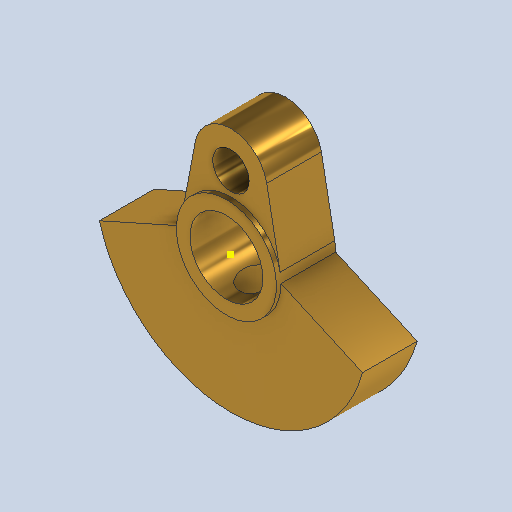
# Autodesk Inventor part: KURBEL PART 8
Saved by Autodesk Inventor 2022 (Build 260153000, 153)
## iProperties
Created: 2020-07-02
Part Number: KURBEL PART 8
Material: Generic
Document SubType Name: Modeling
Designer: Smit Ambardekar
Density: 1 g/cm^3
Appearance: Default
Author: Smit Ambardekar
Autodesk Inventor part; units mm, degrees
ref_plane "YZ Plane" through (0, 0, 0) normal (1, 0, 0) x (0, 1, 0)
ref_plane "XZ Plane" through (0, 0, 0) normal (0, 1, 0) x (-1, 0, 0)
sketch "Sketch1" plane through (0, 0, 0) normal (0, 0, 1) x (1, 0, 0)
  arc A0 (-14.4568, -4) -> (14.4568, -4) centre (0, 0) ccw
  circle A1 centre (0, 0) radius 5.5
  line L0 (0, 0) -> (0, -4)
  line L1 (-5.5, 0) -> (-14.4568, -4)
  line L2 (5.5, 0) -> (14.4568, -4)
  line L3 (0, 0) -> (0, 8)
  circle A2 centre (0, 8) radius 2
  line L4 (-5.4025, 1.0312) -> (-3.9291, 8.75)
  line L5 (3.9291, 8.75) -> (5.4025, 1.0313)
  arc A3 (3.9291, 8.75) -> (-3.9291, 8.75) centre (0, 8) ccw
  line L6 (-2, 14.8661) -> (2, 14.8661)
  line L7 (2, 14.8661) -> (2, -14.8661)
  line L8 (2, -14.8661) -> (-2, -14.8661)
  line L9 (-2, -14.8661) -> (-2, 14.8661)
  line L10 (-2, 14.8661) -> (2, -14.8661) construction
  line L11 (2, 14.8661) -> (-2, -14.8661) construction
  dimension "d0" = 30
  dimension "d1" = 11
  dimension "d2" = 4
  dimension "d3" = 8
  dimension "d4" = 4
  constraints: 24 end point, 9 point on circle, 4 centre point, 4 coincident, 4 tangent, 2 midpoint, 2 parallel, 2 vertical, 1 horizontal, 1 perpendicular
  measures "d0" diameter of A0
  measures "d1" diameter of A1
  measures "d2" distance of L0.start L0.end
  measures "d3" distance of L0.start L3.end
  measures "d4" diameter of A2
extrude "Extrusion1" add sketch "Sketch1" along normal blind 6 contours L1 A1 L9 A0 | L8 A0 | L9 A1 L7 L8 | A1 L9 | L7 A1 L2 A0 | L9 A1 L7 | L4 A3 L9 A1 | L7 A1 | L9 A2 L3 A1 | L7 A3 L5 A1 | A1 L3 A2 L7 | L9 A3 L7 A2
sketch "Sketch2" plane through (0, 0, 6) normal (0, 0, 1) x (1, 0, 0)
  arc A0 (5.5, 0) -> (5.4025, 1.0313) centre (0, 0) ccw projected
  circle A1 centre (0, 0) radius 5.5
  point P0 (5.4025, 1.0313)
  constraints: 1 coincident, 3 other
extrude "Extrusion2" add sketch "Sketch2" along normal blind 0.5
sketch "Sketch3" plane through (0, 0, 6.5) normal (0, 0, 1) x (1, 0, 0)
  point P0 (0, 0)
hole "Hole2" at (0, 0, 6.5) direction (0, 0, -1) diameter 8 end through all
sketch "Sketch4" plane through (0, 0, 6) normal (0, 0, 1) x (1, 0, 0)
  point P0 (0, 0)
ref_plane "Work Plane1" through (-2, -14.8661, 0) normal (0, 1, 0) x (1, 0, 0)
sketch "Sketch5" plane through (-2, -14.8661, 0) normal (0, 1, 0) x (1, 0, 0)
  line L0 (4, -6) -> (0, -6) projected
  line L1 (2, -6) -> (2, -3)
  point P0 (2, 0)
  dimension "d26" = 3
  constraints: 2 end point, 1 midpoint, 1 vertical
  measures "d26" distance of L1.start L1.end
hole "Hole3" at (0, -14.8661, 3) direction (0, 1, 0) diameter 4 depth 11 tip angle 118
sketch "Sketch6" plane through (-2, -14.8661, 0) normal (0, 1, 0) x (1, 0, 0)
  arc A0 (4, -3) -> (0, -3) centre (2, -3) ccw projected
  circle A1 centre (2, -3) radius 2
  point P0 (2, 0)
  constraints: 1 centre point, 1 coincident
hole "Hole4" at (0, -14.8661, 3) direction (0, -1, 0) diameter 4 depth 11 tip angle 118
body "Solid1"
